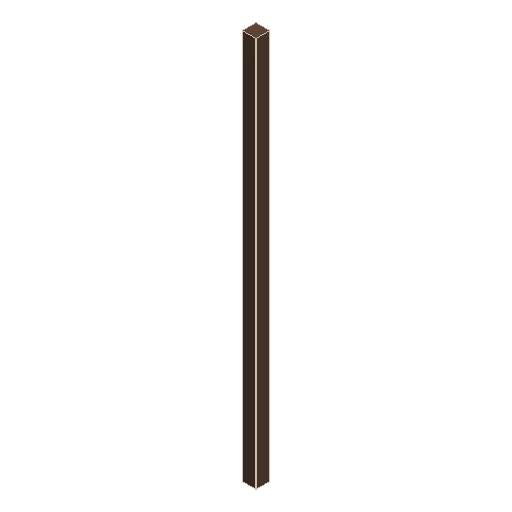
# Autodesk Inventor part: COTS_GENERIC_Balcony_Railing
Saved by Autodesk Inventor 2026 (Build 300175000, 175)
## iProperties
Created: 2025-06-22
Part Number: COTS_GENERIC_Balcony_Railing
Material: Generic
Document SubType Name: Modeling
Designer: User
Density: 1 g/cm^3
Appearance: Bronze - Satin
Author: User
Autodesk Inventor part; units mm, degrees
ref_plane "YZ Plane" through (0, 0, 0) normal (1, 0, 0) x (0, 1, 0)
ref_plane "XZ Plane" through (0, 0, 0) normal (0, 1, 0) x (-1, 0, 0)
ref_plane "XY Plane" through (0, 0, 0) normal (0, 0, 1) x (1, 0, 0)
sketch "Sketch1" plane through (0, 0, 0) normal (0, 1, 0) x (-1, 0, 0)
  line L0 (17.7, 17.7) -> (-17.7, 17.7)
  line L1 (-17.7, 17.7) -> (-17.7, -17.7)
  line L2 (-17.7, -17.7) -> (17.7, -17.7)
  line L3 (17.7, -17.7) -> (17.7, 17.7)
  point P0 (0, 0)
  dimension "d0" = 35.4
  dimension "d1" = 35.4
  dimension "d2" = 17.7
  dimension "d3" = 17.7
  constraints: 8 end point, 2 parallel, 1 horizontal, 1 perpendicular
  measures "d0" distance of L2.end L1.end
  measures "d1" distance of L1.end L0.end
  measures "d2" distance from line of L3 point (0, 0)
  measures "d3" distance from line of L0 point (0, 0)
extrude "Extrusion1" add sketch "Sketch1" along normal blind 1000
fillet "Fillet1" radius 1 4 edges at (17.7, 500, 17.7) (17.7, 500, -17.7) (-17.7, 500, -17.7) (-17.7, 500, 17.7)
equation "\"d2\" = 0.5 * d0"
equation "\"d3\" = 0.5 * d1"
body "Solid1"
